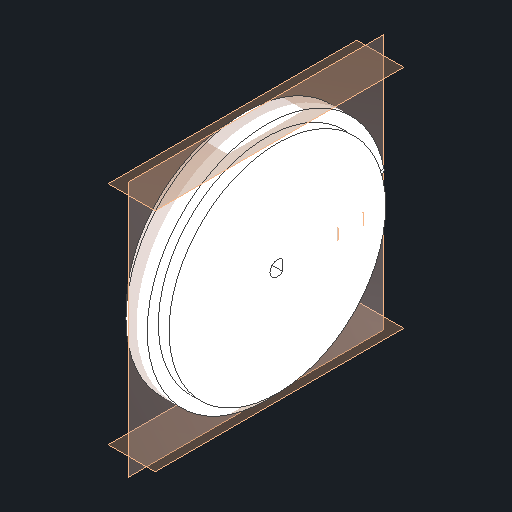
# Autodesk Inventor part: Lock Wheel New Rubber
Saved by Autodesk Inventor 2026.2 (Build 302298000, 298)
## iProperties
Created: 2022-07-23
Part Number: Lock Wheel New Rubber
Material: Generic
Document SubType Name: Modeling
Designer: vandj
Density: 1 g/cm^3
Appearance: Default
Author: vandj
Autodesk Inventor part; units mm, degrees
ref_plane "YZ Plane" through (0, 0, 0) normal (1, 0, 0) x (0, 1, 0)
ref_plane "XY Plane" through (0, 0, 0) normal (0, 0, 1) x (1, 0, 0)
sketch "Sketch1" plane through (0, 0, 0) normal (1, 0, 0) x (0, 1, 0)
  arc A0 (1.1581, -1.06) -> (-1.1581, -1.06) centre (0, 0) ccw
  line L0 (1.1581, -1.06) -> (-1.1581, -1.06)
  circle A1 centre (0, 0) radius 26.5
  constraints: 2 centre point, 2 end point, 2 point on circle, 1 coincident, 1 horizontal
extrude "Extrusion1" add sketch "Sketch1" along normal blind 10
ref_plane "Work Plane1" through (0, 26.5, 0) normal (0, 1, 0) x (-1, 0, 0)
ref_plane "Work Plane2" through (0, -26.5, 0) normal (0, 1, 0) x (-1, 0, 0)
sketch "Sketch6" plane through (10, 0, 0) normal (1, 0, 0) x (0, 0, -1)
  arc A0 (26.4953, 0.5) -> (26.4953, -0.5) centre (0, 0) ccw projected
  line L0 (0, 26.5) -> (0, 27.25)
  arc A1 (26.4953, 0.5) -> (26.4953, -0.5) centre (0, 0) ccw
  circle A2 centre (0, 0) radius 26.5 projected
  circle A3 centre (0, 0) radius 26.5
  circle A4 centre (0, 0) radius 27.25
  dimension "d22" = 0.75
  constraints: 4 point on circle, 2 coincident, 2 end point, 2 vertical alignment, 1 centre point, 1 vertical, 4 other
  measures "d22" distance of L0.start L0.end
extrude "Extrusion6" add sketch "Sketch6" against normal blind 1
ref_plane "Work Plane3" through (5, 0, 0) normal (1, 0, 0) x (0, 0, -1)
mirror "Mirror1" about plane through (5, 0, 0) normal (1, 0, 0) of "Extrusion6"
sketch "Sketch7" plane through (0, -1.1581, -1.06) normal (0, 0, 1) x (1, 0, 0)
  line L0 (1, 27.6581) -> (9, 27.6581) projected
  line L1 (5, 27.6581) -> (5, -25.3419)
  line L2 (1, -25.3419) -> (9, -25.3419) projected
  line L3 (10, 2.3163) -> (10, 0) projected
  line L4 (10, 1.1581) -> (-0.1429, 1.1581)
  circle A0 centre (5, 1.1581) radius 1.8
  dimension "d28" = 3.6
  constraints: 4 end point, 3 midpoint, 1 centre point, 1 horizontal
  measures "d28" diameter of A0
extrude "Extrusion7" cut sketch "Sketch7" against normal blind 13
ref_plane "Work Plane4" through (10, -1.1581, -14.06) normal (0, 0, 1) x (1, 0, 0)
sketch "Sketch8" plane through (10, -1.1581, -14.06) normal (0, 0, 1) x (1, 0, 0)
  arc A0 (-6.3779, 0) -> (-3.6221, 0) centre (-5, 1.1581) ccw projected
  circle A1 centre (-5, 1.1581) radius 2.05
  point P0 (-10, 1.1581)
  dimension "d32" = 4.1
  constraints: 1 centre point, 1 coincident
  measures "d32" diameter of A1
extrude "Extrusion8" cut sketch "Sketch8" against normal blind 6
ref_plane "Work Plane5" through (10, -1.1581, -20.06) normal (0, 0, 1) x (1, 0, 0)
sketch "Sketch10" plane through (10, 0, 0) normal (1, 0, 0) x (0, 0, -1)
  circle A0 centre (0, 0) radius 27.25 projected
  circle A1 centre (0, 0) radius 1.75
  line L0 (1.2405, 1.2351) -> (1.2405, -1.2351)
  arc A2 (1.2405, 1.2351) -> (1.2405, -1.2351) centre (0, 0) ccw
  point P0 (1.2405, -1.2344)
  point P1 (1.2405, 1.2344)
  dimension "d40" = 3.5
  constraints: 2 centre point, 2 end point, 2 point on circle, 1 coincident
  measures "d40" diameter of A1
extrude "Extrusion10" cut sketch "Sketch10" against normal blind 15.575 contours L0 A1 picked at (0.3435, -0.5243)
sketch "Sketch11" plane through (10, 0, 0) normal (1, 0, 0) x (0, 0, -1)
  circle A0 centre (0, 0) radius 27.25 projected
  arc A1 (1.2405, 1.2344) -> (1.2405, -1.2344) centre (0, 0) ccw projected
  circle A2 centre (0, 0) radius 25.4
  dimension "d44" = 50.8
  constraints: 1 centre point, 1 coincident
  measures "d44" diameter of A2
extrude "Extrusion11" cut sketch "Sketch11" against normal blind 10
sketch "Sketch12" plane through (5, 0, 0) normal (1, 0, 0) x (0, 0, -1)
  circle A0 centre (0, 0) radius 28
  circle A1 centre (0, 0) radius 25.4
  dimension "d45" = 56
  constraints: 2 centre point, 2 coincident
  measures "d45" diameter of A0
extrude "Extrusion12" add sketch "Sketch12" along normal mid plane 5
sketch "Sketch9" plane through (10, -1.1581, -20.06) normal (0, 0, 1) x (1, 0, 0)
  circle A0 centre (-5, 1.1581) radius 1.8 projected
  circle A1 centre (-5, 1.1581) radius 4.3333
  circle A2 centre (-5, 1.1581) radius 2.05 projected
  circle A3 centre (-5, 1.1581) radius 3.25
  point P0 (-10, 1.1581)
  dimension "d41" = 6.5
  constraints: 2 centre point, 2 coincident
  measures "d41" diameter of A3
extrude "Extrusion9" cut sketch "Sketch9" against normal blind 16.225 contours A0 | A2 | A3
fillet "Fillet1" radius 2 4 edges at (2.5, 2.0767, -26.6189) (2.5, -2.0767, -26.6189) (7.5, -2.0767, -26.6189) (7.5, 2.0767, -26.6189)
body "Solid1"
